Autodesk Fusion 360 part; units mm, degrees
(part 12 of 14)
  arc A3353 (43.5673, 5.334) -> (44.0627, 5.334) centre (43.815, 5.334) ccw
  line L5719 (41.91, 3.8608) -> (50.8, 3.8608)
  line L5720 (43.815, 5.08) -> (43.815, 5.588)
  line L5721 (43.561, 5.334) -> (44.069, 5.334)
  line L5722 (43.815, 5.08) -> (43.815, 5.588)
  arc A3354 (63.8873, 6.223) -> (64.3827, 6.223) centre (64.135, 6.223) ccw
  line L5723 (41.91, 6.8072) -> (41.91, 3.8608)
  line L5724 (64.389, 6.223) -> (63.881, 6.223)
  arc A3355 (64.3827, 6.223) -> (63.8873, 6.223) centre (64.135, 6.223) ccw
  arc A3356 (43.5673, 5.334) -> (44.0627, 5.334) centre (43.815, 5.334) ccw
  line L5725 (64.389, 6.223) -> (63.881, 6.223)
  arc A3357 (63.8873, 6.223) -> (64.3827, 6.223) centre (64.135, 6.223) ccw
  line L5726 (64.135, 6.477) -> (64.135, 5.969)
  line L5727 (64.135, 6.477) -> (64.135, 5.969)
  line L5728 (43.815, 5.08) -> (43.815, 5.588)
  arc A3358 (64.135, 6.477) -> (64.135, 5.969) centre (64.135, 6.223) ccw
  arc A3359 (43.5673, 5.334) -> (44.0627, 5.334) centre (43.815, 5.334) ccw
  line L5729 (43.561, 5.334) -> (44.069, 5.334)
  line L5730 (50.8, 3.8608) -> (50.8, 6.8072)
  line L5731 (43.561, 5.334) -> (44.069, 5.334)
  line L5732 (43.815, 5.08) -> (43.815, 5.588)
  arc A3360 (64.3827, 6.223) -> (63.8873, 6.223) centre (64.135, 6.223) ccw
  arc A3361 (43.5673, 5.334) -> (44.0627, 5.334) centre (43.815, 5.334) ccw
  arc A3362 (46.1073, 5.334) -> (46.6026, 5.334) centre (46.355, 5.334) ccw
  arc A3363 (46.355, 4.9403) -> (46.355, 5.7277) centre (46.355, 5.334) ccw
  arc A3364 (46.1073, 5.334) -> (46.6026, 5.334) centre (46.355, 5.334) ccw
  arc A3365 (46.6026, 5.334) -> (46.1073, 5.334) centre (46.355, 5.334) ccw
  line L5733 (46.355, 5.08) -> (46.355, 5.588)
  arc A3366 (46.355, 5.7277) -> (46.355, 4.9403) centre (46.355, 5.334) ccw
  arc A3367 (44.0627, 5.334) -> (43.5673, 5.334) centre (43.815, 5.334) ccw
  line L5734 (46.355, 5.08) -> (46.355, 5.588)
  arc A3368 (46.355, 4.9403) -> (46.355, 5.7277) centre (46.355, 5.334) ccw
  line L5735 (46.355, 5.08) -> (46.355, 5.588)
  arc A3369 (44.0627, 5.334) -> (43.5673, 5.334) centre (43.815, 5.334) ccw
  arc A3370 (46.355, 5.588) -> (46.355, 5.08) centre (46.355, 5.334) ccw
  arc A3371 (49.1427, 5.334) -> (48.6473, 5.334) centre (48.895, 5.334) ccw
  line L5736 (46.355, 5.08) -> (46.355, 5.588)
  line L5737 (43.815, 5.08) -> (43.815, 5.588)
  arc A3372 (46.1073, 5.334) -> (46.6026, 5.334) centre (46.355, 5.334) ccw
  line L5738 (46.355, 5.08) -> (46.355, 5.588)
  arc A3373 (46.1073, 5.334) -> (46.6026, 5.334) centre (46.355, 5.334) ccw
  line L5739 (43.815, 5.08) -> (43.815, 5.588)
  arc A3374 (46.6026, 5.334) -> (46.1073, 5.334) centre (46.355, 5.334) ccw
  arc A3375 (44.0627, 5.334) -> (43.5673, 5.334) centre (43.815, 5.334) ccw
  line L5740 (43.815, 5.08) -> (43.815, 5.588)
  arc A3376 (44.0627, 5.334) -> (43.5673, 5.334) centre (43.815, 5.334) ccw
  arc A3377 (48.6473, 5.334) -> (49.1427, 5.334) centre (48.895, 5.334) ccw
  arc A3378 (49.1427, 5.334) -> (48.6473, 5.334) centre (48.895, 5.334) ccw
  arc A3379 (46.6026, 5.334) -> (46.1073, 5.334) centre (46.355, 5.334) ccw
  arc A3380 (46.1073, 5.334) -> (46.6026, 5.334) centre (46.355, 5.334) ccw
  arc A3381 (46.355, 4.9403) -> (46.355, 5.7277) centre (46.355, 5.334) ccw
  arc A3382 (48.6473, 5.334) -> (49.1427, 5.334) centre (48.895, 5.334) ccw
  arc A3383 (46.1073, 5.334) -> (46.6026, 5.334) centre (46.355, 5.334) ccw
  arc A3384 (46.6026, 5.334) -> (46.1073, 5.334) centre (46.355, 5.334) ccw
  arc A3385 (46.6026, 5.334) -> (46.1073, 5.334) centre (46.355, 5.334) ccw
  arc A3386 (46.355, 5.08) -> (46.355, 5.588) centre (46.355, 5.334) ccw
  line L5741 (48.895, 5.08) -> (48.895, 5.588)
  line L5742 (46.355, 5.08) -> (46.355, 5.588)
  arc A3387 (46.6026, 5.334) -> (46.1073, 5.334) centre (46.355, 5.334) ccw
  line L5743 (46.101, 5.334) -> (46.609, 5.334)
  line L5744 (46.101, 5.334) -> (46.609, 5.334)
  line L5745 (46.101, 5.334) -> (46.609, 5.334)
  line L5746 (46.101, 5.334) -> (46.609, 5.334)
  arc A3388 (46.355, 5.7277) -> (46.355, 4.9403) centre (46.355, 5.334) ccw
  line L5747 (43.815, 5.08) -> (43.815, 5.588)
  arc A3389 (46.1073, 5.334) -> (46.6026, 5.334) centre (46.355, 5.334) ccw
  arc A3390 (46.355, 4.9403) -> (46.355, 5.7277) centre (46.355, 5.334) ccw
  arc A3391 (44.0627, 5.334) -> (43.5673, 5.334) centre (43.815, 5.334) ccw
  line L5748 (46.355, 5.08) -> (46.355, 5.588)
  arc A3392 (48.6473, 5.334) -> (49.1427, 5.334) centre (48.895, 5.334) ccw
  line L5749 (46.101, 5.334) -> (46.609, 5.334)
  line L5750 (46.101, 5.334) -> (46.609, 5.334)
  arc A3393 (46.6026, 5.334) -> (46.1073, 5.334) centre (46.355, 5.334) ccw
  arc A3394 (46.355, 5.7277) -> (46.355, 4.9403) centre (46.355, 5.334) ccw
  line L5751 (46.355, 5.08) -> (46.355, 5.588)
  arc A3395 (46.6026, 5.334) -> (46.1073, 5.334) centre (46.355, 5.334) ccw
  line L5752 (48.895, 5.08) -> (48.895, 5.588)
  arc A3396 (46.355, 4.9403) -> (46.355, 5.7277) centre (46.355, 5.334) ccw
  line L5753 (46.101, 5.334) -> (46.609, 5.334)
  line L5754 (46.101, 5.334) -> (46.609, 5.334)
  line L5755 (43.0276, 5.334) -> (44.6024, 5.334)
  arc A3397 (46.355, 5.7277) -> (46.355, 4.9403) centre (46.355, 5.334) ccw
  line L5756 (46.355, 5.08) -> (46.355, 5.588)
  arc A3398 (46.6026, 5.334) -> (46.1073, 5.334) centre (46.355, 5.334) ccw
  line L5757 (46.101, 5.334) -> (46.609, 5.334)
  line L5758 (48.641, 5.334) -> (49.149, 5.334)
  arc A3399 (46.1073, 5.334) -> (46.6026, 5.334) centre (46.355, 5.334) ccw
  arc A3400 (48.895, 4.9403) -> (48.895, 5.7277) centre (48.895, 5.334) ccw
  line L5759 (30.607, 2.667) -> (39.116, 2.667)
  arc A3401 (48.6473, 5.334) -> (49.1427, 5.334) centre (48.895, 5.334) ccw
  line L5760 (48.895, 5.08) -> (48.895, 5.588)
  line L5761 (48.895, 5.08) -> (48.895, 5.588)
  arc A3402 (46.6026, 5.334) -> (46.1073, 5.334) centre (46.355, 5.334) ccw
  arc A3403 (46.355, 5.7277) -> (46.355, 4.9403) centre (46.355, 5.334) ccw
  line L5762 (48.641, 5.334) -> (49.149, 5.334)
  arc A3404 (49.1427, 5.334) -> (48.6473, 5.334) centre (48.895, 5.334) ccw
  line L5763 (39.116, 2.667) -> (39.116, 7.747)
  arc A3405 (48.895, 5.588) -> (48.895, 5.08) centre (48.895, 5.334) ccw
  line L5764 (48.895, 5.08) -> (48.895, 5.588)
  arc A3406 (48.6473, 5.334) -> (49.1427, 5.334) centre (48.895, 5.334) ccw
  arc A3407 (49.1427, 5.334) -> (48.6473, 5.334) centre (48.895, 5.334) ccw
  arc A3408 (49.1427, 5.334) -> (48.6473, 5.334) centre (48.895, 5.334) ccw
  line L5765 (48.895, 5.08) -> (48.895, 5.588)
  arc A3409 (48.6473, 5.334) -> (49.1427, 5.334) centre (48.895, 5.334) ccw
  arc A3410 (48.895, 5.7277) -> (48.895, 4.9403) centre (48.895, 5.334) ccw
  arc A3411 (49.1427, 5.334) -> (48.6473, 5.334) centre (48.895, 5.334) ccw
  line L5766 (25.256, 2.707) -> (25.556, 3.407)
  arc A3412 (48.895, 4.9403) -> (48.895, 5.7277) centre (48.895, 5.334) ccw
  line L5767 (48.895, 5.08) -> (48.895, 5.588)
  arc A3413 (48.6473, 5.334) -> (49.1427, 5.334) centre (48.895, 5.334) ccw
  line L5768 (26.416, 6.007) -> (26.416, 8.407)
  line L5769 (26.416, 6.007) -> (26.416, 8.407)
  line L5770 (27.686, 6.007) -> (27.686, 8.407)
  arc A3414 (49.1427, 5.334) -> (48.6473, 5.334) centre (48.895, 5.334) ccw
  line L5771 (28.956, 2.007) -> (28.956, 4.407)
  line L5772 (48.641, 5.334) -> (49.149, 5.334)
  line L5773 (48.641, 5.334) -> (49.149, 5.334)
  line L5774 (48.641, 5.334) -> (49.149, 5.334)
  line L5775 (48.641, 5.334) -> (49.149, 5.334)
  arc A3415 (48.895, 5.7277) -> (48.895, 4.9403) centre (48.895, 5.334) ccw
  line L5776 (27.305, 7.747) -> (25.146, 7.747)
  arc A3416 (48.895, 4.9403) -> (48.895, 5.7277) centre (48.895, 5.334) ccw
  arc A3417 (48.895, 5.7277) -> (48.895, 4.9403) centre (48.895, 5.334) ccw
  arc A3418 (49.1427, 5.334) -> (48.6473, 5.334) centre (48.895, 5.334) ccw
  line L5777 (48.895, 5.08) -> (48.895, 5.588)
  arc A3419 (48.6473, 5.334) -> (49.1427, 5.334) centre (48.895, 5.334) ccw
  arc A3420 (48.895, 5.7277) -> (48.895, 4.9403) centre (48.895, 5.334) ccw
  arc A3421 (46.1073, 5.334) -> (46.6026, 5.334) centre (46.355, 5.334) ccw
  arc A3422 (46.1073, 5.334) -> (46.6026, 5.334) centre (46.355, 5.334) ccw
  line L5778 (48.641, 5.334) -> (49.149, 5.334)
  line L5779 (46.355, 5.08) -> (46.355, 5.588)
  line L5780 (48.895, 5.08) -> (48.895, 5.588)
  line L5781 (48.641, 5.334) -> (49.149, 5.334)
  arc A3423 (49.1427, 5.334) -> (48.6473, 5.334) centre (48.895, 5.334) ccw
  arc A3424 (48.895, 4.9403) -> (48.895, 5.7277) centre (48.895, 5.334) ccw
  arc A3425 (48.895, 4.9403) -> (48.895, 5.7277) centre (48.895, 5.334) ccw
  line L5782 (46.101, 5.334) -> (46.609, 5.334)
  line L5783 (39.116, 7.747) -> (30.607, 7.747)
  line L5784 (48.641, 5.334) -> (49.149, 5.334)
  arc A3426 (49.1427, 5.334) -> (48.6473, 5.334) centre (48.895, 5.334) ccw
  line L5785 (25.146, 7.747) -> (25.146, 2.667)
  line L5786 (25.556, 3.407) -> (25.856, 2.707)
  arc A3427 (48.895, 5.08) -> (48.895, 5.588) centre (48.895, 5.334) ccw
  line L5787 (25.146, 2.667) -> (27.305, 2.667)
  line L5788 (48.641, 5.334) -> (49.149, 5.334)
  arc A3428 (48.6473, 5.334) -> (49.1427, 5.334) centre (48.895, 5.334) ccw
  arc A3429 (48.6473, 5.334) -> (49.1427, 5.334) centre (48.895, 5.334) ccw
  arc A3430 (48.895, 5.7277) -> (48.895, 4.9403) centre (48.895, 5.334) ccw
  line L5789 (28.067, 2.667) -> (29.845, 2.667)
  line L5790 (48.895, 5.08) -> (48.895, 5.588)
  line L5791 (29.845, 7.747) -> (28.067, 7.747)
  line L5792 (36.576, 6.007) -> (36.576, 8.407)
  line L5793 (86.233, 32.893) -> (86.233, 36.703)
  line L5794 (32.766, 6.007) -> (32.766, 8.407)
  arc A3431 (85.9944, 37.338) -> (86.4716, 37.338) centre (86.233, 37.338) ccw
  line L5795 (85.344, 37.211) -> (85.852, 37.211)
  line L5796 (30.226, 2.007) -> (30.226, 4.407)
  line L5797 (34.036, 2.007) -> (34.036, 4.407)
  line L5798 (86.233, 36.703) -> (82.423, 36.703)
  line L5799 (82.804, 32.385) -> (83.312, 32.385)
  line L5800 (12.2702, 55.37) -> (18.8702, 55.37)
  line L5801 (30.226, 2.007) -> (30.226, 4.407)
  line L5802 (31.496, 2.007) -> (31.496, 4.407)
  line L5803 (30.226, 2.007) -> (30.226, 4.407)
  line L5804 (82.804, 37.211) -> (83.312, 37.211)
  line L5805 (34.036, 2.007) -> (34.036, 4.407)
  line L5806 (27.686, 6.007) -> (27.686, 8.407)
  line L5807 (35.306, 2.007) -> (35.306, 4.407)
  line L5808 (27.686, 2.007) -> (27.686, 4.407)
  line L5809 (35.306, 6.007) -> (35.306, 8.407)
  line L5810 (31.496, 6.007) -> (31.496, 8.407)
  line L5811 (35.306, 6.007) -> (35.306, 8.407)
  line L5812 (32.766, 6.007) -> (32.766, 8.407)
  line L5813 (27.686, 2.007) -> (27.686, 4.407)
  line L5814 (32.766, 2.007) -> (32.766, 4.407)
  line L5815 (34.036, 6.007) -> (34.036, 8.407)
  line L5816 (37.846, 6.007) -> (37.846, 8.407)
  line L5817 (28.956, 6.007) -> (28.956, 8.407)
  line L5818 (18.8702, 48.77) -> (12.2702, 48.77)
  line L5819 (27.686, 2.007) -> (27.686, 4.407)
  line L5820 (34.036, 6.007) -> (34.036, 8.407)
  line L5821 (82.804, 37.211) -> (83.312, 37.211)
  line L5822 (27.686, 6.007) -> (27.686, 8.407)
  line L5823 (34.036, 6.007) -> (34.036, 8.407)
  line L5824 (82.804, 32.385) -> (83.312, 32.385)
  line L5825 (84.074, 37.211) -> (84.582, 37.211)
  line L5826 (36.576, 2.007) -> (36.576, 4.407)
  line L5827 (35.306, 2.007) -> (35.306, 4.407)
  line L5828 (36.576, 6.007) -> (36.576, 8.407)
  line L5829 (28.956, 6.007) -> (28.956, 8.407)
  line L5830 (31.496, 6.007) -> (31.496, 8.407)
  line L5831 (32.766, 6.007) -> (32.766, 8.407)
  line L5832 (28.956, 2.007) -> (28.956, 4.407)
  line L5833 (36.576, 2.007) -> (36.576, 4.407)
  line L5834 (26.416, 2.007) -> (26.416, 4.407)
  line L5835 (31.496, 2.007) -> (31.496, 4.407)
  line L5836 (26.416, 2.007) -> (26.416, 4.407)
  line L5837 (30.226, 6.007) -> (30.226, 8.407)
  line L5838 (26.416, 6.007) -> (26.416, 8.407)
  line L5839 (28.956, 6.007) -> (28.956, 8.407)
  line L5840 (32.766, 2.007) -> (32.766, 4.407)
  line L5841 (30.226, 6.007) -> (30.226, 8.407)
  line L5842 (37.846, 2.007) -> (37.846, 4.407)
  line L5843 (31.496, 2.007) -> (31.496, 4.407)
  line L5844 (36.576, 2.007) -> (36.576, 4.407)
  line L5845 (34.036, 2.007) -> (34.036, 4.407)
  line L5846 (30.226, 6.007) -> (30.226, 8.407)
  line L5847 (26.416, 2.007) -> (26.416, 4.407)
  line L5848 (35.306, 2.007) -> (35.306, 4.407)
  line L5849 (36.576, 6.007) -> (36.576, 8.407)
  line L5850 (31.496, 6.007) -> (31.496, 8.407)
  line L5851 (32.766, 2.007) -> (32.766, 4.407)
  line L5852 (35.306, 6.007) -> (35.306, 8.407)
  line L5853 (85.852, 33.909) -> (85.852, 35.687)
  line L5854 (28.956, 2.007) -> (28.956, 4.407)
  line L5855 (86.106, 22.352) -> (82.296, 22.352)
  line L5856 (68.834, 38.735) -> (69.342, 38.735)
  line L5857 (82.804, 32.385) -> (83.312, 32.385)
  line L5858 (82.296, 22.352) -> (82.296, 18.542)
  line L5859 (70.104, 38.735) -> (70.612, 38.735)
  line L5860 (82.296, 18.542) -> (86.106, 18.542)
  line L5861 (18.7702, 54.27) -> (12.3702, 54.27)
  line L5862 (18.7702, 49.87) -> (12.3702, 49.87)
  arc A3432 (72.5016, 38.862) -> (72.0244, 38.862) centre (72.263, 38.862) ccw
  line L5863 (82.677, 21.336) -> (82.677, 19.558)
  line L5864 (83.185, 18.034) -> (82.677, 18.034)
  arc A3433 (86.4716, 37.338) -> (85.9944, 37.338) centre (86.233, 37.338) ccw
  line L5865 (84.074, 37.211) -> (84.582, 37.211)
  line L5866 (82.804, 35.687) -> (82.804, 33.909)
  line L5867 (72.263, 38.227) -> (68.453, 38.227)
  line L5868 (68.453, 34.417) -> (72.263, 34.417)
  line L5869 (71.374, 38.735) -> (71.882, 38.735)
  line L5870 (71.374, 33.909) -> (71.882, 33.909)
  arc A3434 (82.5346, 17.907) -> (82.0574, 17.907) centre (82.296, 17.907) ccw
  line L5871 (72.263, 34.417) -> (72.263, 38.227)
  line L5872 (82.804, 37.211) -> (83.312, 37.211)
  line L5873 (68.834, 16.764) -> (71.882, 16.764)
  line L5874 (71.882, 18.542) -> (68.834, 18.542)
  line L5875 (85.725, 18.034) -> (85.217, 18.034)
  line L5876 (71.882, 16.764) -> (71.882, 18.542)
  line L5877 (83.185, 22.86) -> (82.677, 22.86)
  line L5878 (37.846, 6.007) -> (37.846, 8.407)
  line L5879 (83.185, 18.034) -> (82.677, 18.034)
  line L5880 (68.834, 33.909) -> (69.342, 33.909)
  line L5881 (85.852, 35.687) -> (82.804, 35.687)
  line L5882 (85.344, 32.385) -> (85.852, 32.385)
  line L5883 (85.344, 32.385) -> (85.852, 32.385)
  line L5884 (82.423, 36.703) -> (82.423, 32.893)
  line L5885 (18.8702, 55.37) -> (18.8702, 48.77)
  line L5886 (84.074, 37.211) -> (84.582, 37.211)
  line L5887 (71.882, 37.211) -> (68.834, 37.211)
  line L5888 (71.374, 38.735) -> (71.882, 38.735)
  line L5889 (82.804, 33.909) -> (85.852, 33.909)
  line L5890 (70.104, 38.735) -> (70.612, 38.735)
  line L5891 (85.344, 32.385) -> (85.852, 32.385)
  line L5892 (18.7702, 54.27) -> (12.3702, 54.27)
  line L5893 (70.104, 38.735) -> (70.612, 38.735)
  line L5894 (37.846, 2.007) -> (37.846, 4.407)
  line L5895 (71.882, 35.433) -> (71.882, 37.211)
  line L5896 (68.834, 33.909) -> (69.342, 33.909)
  line L5897 (68.453, 38.227) -> (68.453, 34.417)
  line L5898 (71.374, 33.909) -> (71.882, 33.909)
  line L5899 (18.7702, 49.87) -> (12.3702, 49.87)
  arc A3435 (72.0244, 38.862) -> (72.5016, 38.862) centre (72.263, 38.862) ccw
  line L5900 (82.423, 32.893) -> (86.233, 32.893)
  line L5901 (37.846, 2.007) -> (37.846, 4.407)
  line L5902 (18.7702, 49.87) -> (12.3702, 49.87)
  line L5903 (68.834, 38.735) -> (69.342, 38.735)
  line L5904 (18.7702, 54.27) -> (12.3702, 54.27)
  line L5905 (37.846, 6.007) -> (37.846, 8.407)
  line L5906 (85.344, 37.211) -> (85.852, 37.211)
  line L5907 (68.834, 38.735) -> (69.342, 38.735)
  line L5908 (12.2702, 48.77) -> (12.2702, 55.37)
  line L5909 (85.344, 37.211) -> (85.852, 37.211)
  line L5910 (68.834, 37.211) -> (68.834, 35.433)
  line L5911 (71.374, 33.909) -> (71.882, 33.909)
  line L5912 (68.834, 33.909) -> (69.342, 33.909)
  line L5913 (71.374, 38.735) -> (71.882, 38.735)
  line L5914 (68.834, 35.433) -> (71.882, 35.433)
  line L5915 (9.652, 22.6974) -> (9.652, 24.1198)
  line L5916 (71.882, 15.24) -> (71.374, 15.24)
  line L5917 (7.659, 22.7336) -> (7.659, 24.0836)
  line L5918 (9.359, 22.7336) -> (9.359, 24.0836)
  line L5919 (69.342, 20.066) -> (68.834, 20.066)
  line L5920 (7.409, 24.1336) -> (7.409, 22.6836)
  line L5921 (85.725, 22.86) -> (85.217, 22.86)
  line L5922 (84.455, 18.034) -> (83.947, 18.034)
  line L5923 (71.882, 20.066) -> (71.374, 20.066)
  line L5924 (83.185, 22.86) -> (82.677, 22.86)
  line L5925 (7.366, 24.1198) -> (7.366, 22.6974)
  line L5926 (5.3823, 40.6654) -> (5.3823, 42.9514)
  line L5927 (85.725, 18.034) -> (85.217, 18.034)
  line L5928 (9.652, 24.1198) -> (7.366, 24.1198)
  line L5929 (3.9599, 42.9514) -> (3.9599, 40.6654)
  line L5930 (3.9599, 40.6654) -> (5.3823, 40.6654)
  line L5931 (82.677, 19.558) -> (85.725, 19.558)
  line L5932 (85.725, 18.034) -> (85.217, 18.034)
  line L5933 (5.3961, 42.9084) -> (3.9461, 42.9084)
  line L5934 (70.612, 15.24) -> (70.104, 15.24)
  line L5935 (9.652, 24.1198) -> (7.366, 24.1198)
  line L5936 (86.106, 18.542) -> (86.106, 22.352)
  line L5937 (71.882, 20.066) -> (71.374, 20.066)
  line L5938 (71.882, 15.24) -> (71.374, 15.24)
  line L5939 (7.366, 24.1198) -> (7.366, 22.6974)
  line L5940 (69.342, 20.066) -> (68.834, 20.066)
  line L5941 (71.882, 20.066) -> (71.374, 20.066)
  line L5942 (7.366, 22.6974) -> (9.652, 22.6974)
  line L5943 (9.359, 22.7336) -> (9.359, 24.0836)
  line L5944 (7.659, 22.7336) -> (7.659, 24.0836)
  line L5945 (9.609, 24.1336) -> (7.409, 24.1336)
  line L5946 (9.652, 22.6974) -> (9.652, 24.1198)
  line L5947 (7.366, 22.6974) -> (9.652, 22.6974)
  line L5948 (5.3961, 40.7084) -> (5.3961, 42.9084)
  line L5949 (85.725, 21.336) -> (82.677, 21.336)
  line L5950 (9.359, 22.7336) -> (9.359, 24.0836)
  line L5951 (3.9461, 40.7084) -> (5.3961, 40.7084)
  line L5952 (3.9461, 42.9084) -> (3.9461, 40.7084)
  line L5953 (7.659, 22.7336) -> (7.659, 24.0836)
  line L5954 (68.453, 19.558) -> (68.453, 15.748)
  line L5955 (84.455, 18.034) -> (83.947, 18.034)
  arc A3436 (68.2144, 15.113) -> (68.6916, 15.113) centre (68.453, 15.113) ccw
  line L5956 (85.725, 22.86) -> (85.217, 22.86)
  line L5957 (69.342, 15.24) -> (68.834, 15.24)
  arc A3437 (82.0574, 17.907) -> (82.5346, 17.907) centre (82.296, 17.907) ccw
  line L5958 (84.455, 18.034) -> (83.947, 18.034)
  line L5959 (69.342, 15.24) -> (68.834, 15.24)
  line L5960 (85.725, 22.86) -> (85.217, 22.86)
  line L5961 (85.725, 19.558) -> (85.725, 21.336)
  line L5962 (72.263, 15.748) -> (72.263, 19.558)
  arc A3438 (68.6916, 15.113) -> (68.2144, 15.113) centre (68.453, 15.113) ccw
  line L5963 (72.263, 19.558) -> (68.453, 19.558)
  line L5964 (68.453, 15.748) -> (72.263, 15.748)
  line L5965 (83.185, 22.86) -> (82.677, 22.86)
  line L5966 (83.185, 18.034) -> (82.677, 18.034)
  line L5967 (7.409, 22.6836) -> (9.609, 22.6836)
  line L5968 (71.882, 15.24) -> (71.374, 15.24)
  line L5969 (68.834, 18.542) -> (68.834, 16.764)
  line L5970 (9.609, 22.6836) -> (9.609, 24.1336)
  line L5971 (5.3823, 42.9514) -> (3.9599, 42.9514)
  line L5972 (70.612, 15.24) -> (70.104, 15.24)
  line L5973 (70.612, 15.24) -> (70.104, 15.24)
  line L5974 (69.342, 20.066) -> (68.834, 20.066)
  line L5975 (69.342, 15.24) -> (68.834, 15.24)
  arc A3439 (93.345, 58.039) -> (93.345, 58.801) centre (93.345, 58.42) ccw
  arc A3440 (93.0973, 58.42) -> (93.5927, 58.42) centre (93.345, 58.42) ccw
  arc A3441 (93.345, 58.801) -> (93.345, 58.039) centre (93.345, 58.42) ccw
  arc A3442 (93.345, 58.801) -> (93.345, 58.039) centre (93.345, 58.42) ccw
  arc A3443 (74.4157, 6.858) -> (73.9203, 6.858) centre (74.168, 6.858) ccw
  line L5976 (23.218, 39.551) -> (16.818, 39.551)
  arc A3444 (93.5927, 58.42) -> (93.0973, 58.42) centre (93.345, 58.42) ccw
  line L5977 (93.091, 58.42) -> (93.599, 58.42)
  line L5978 (93.091, 58.42) -> (93.599, 58.42)
  line L5979 (93.345, 58.166) -> (93.345, 58.674)
  line L5980 (16.718, 45.051) -> (23.318, 45.051)
  arc A3445 (74.168, 7.493) -> (74.168, 6.223) centre (74.168, 6.858) ccw
  line L5981 (93.345, 58.166) -> (93.345, 58.674)
  arc A3446 (74.4157, 6.858) -> (73.9203, 6.858) centre (74.168, 6.858) ccw
  arc A3447 (93.345, 59.055) -> (93.345, 57.785) centre (93.345, 58.42) ccw
  line L5982 (93.091, 58.42) -> (93.599, 58.42)
  arc A3448 (94.615, 58.42) -> (92.075, 58.42) centre (93.345, 58.42) ccw
  arc A3449 (93.0973, 58.42) -> (93.5927, 58.42) centre (93.345, 58.42) ccw
  line L5983 (93.345, 58.166) -> (93.345, 58.674)
  arc A3450 (94.5919, 58.42) -> (92.0981, 58.42) centre (93.345, 58.42) ccw
  line L5984 (93.345, 58.166) -> (93.345, 58.674)
  line L5985 (3.9599, 42.9514) -> (3.9599, 40.6654)
  line L5986 (5.3461, 40.9584) -> (3.9961, 40.9584)
  line L5987 (93.091, 58.42) -> (93.599, 58.42)
  line L5988 (93.091, 58.42) -> (93.599, 58.42)
  line L5989 (93.345, 58.166) -> (93.345, 58.674)
  arc A3451 (93.5927, 58.42) -> (93.0973, 58.42) centre (93.345, 58.42) ccw
  arc A3452 (72.9211, 6.858) -> (75.4149, 6.858) centre (74.168, 6.858) ccw
  arc A3453 (93.5927, 58.42) -> (93.0973, 58.42) centre (93.345, 58.42) ccw
  line L5990 (5.3461, 42.6584) -> (3.9961, 42.6584)
  line L5991 (5.3461, 40.9584) -> (3.9961, 40.9584)
  line L5992 (23.218, 39.551) -> (16.818, 39.551)
  line L5993 (23.218, 39.551) -> (16.818, 39.551)
  arc A3454 (93.0973, 58.42) -> (93.5927, 58.42) centre (93.345, 58.42) ccw
  arc A3455 (93.0973, 58.42) -> (93.5927, 58.42) centre (93.345, 58.42) ccw
  arc A3456 (92.0981, 58.42) -> (94.5919, 58.42) centre (93.345, 58.42) ccw
  line L5994 (74.168, 7.112) -> (74.168, 6.604)
  line L5995 (5.3461, 40.9584) -> (3.9961, 40.9584)
  arc A3457 (92.075, 58.42) -> (94.615, 58.42) centre (93.345, 58.42) ccw
  arc A3458 (93.5927, 58.42) -> (93.0973, 58.42) centre (93.345, 58.42) ccw
  line L5996 (23.218, 43.951) -> (16.818, 43.951)
  arc A3459 (93.0973, 58.42) -> (93.5927, 58.42) centre (93.345, 58.42) ccw
  line L5997 (93.345, 58.166) -> (93.345, 58.674)
  line L5998 (5.3823, 42.9514) -> (3.9599, 42.9514)
  line L5999 (5.3823, 40.6654) -> (5.3823, 42.9514)
  line L6000 (5.3461, 42.6584) -> (3.9961, 42.6584)
  line L6001 (5.3461, 42.6584) -> (3.9961, 42.6584)
  line L6002 (23.218, 43.951) -> (16.818, 43.951)
  line L6003 (23.218, 43.951) -> (16.818, 43.951)
  line L6004 (74.422, 6.858) -> (73.914, 6.858)
  line L6005 (16.718, 38.451) -> (16.718, 45.051)
  line L6006 (23.318, 38.451) -> (16.718, 38.451)
  line L6007 (3.9599, 40.6654) -> (5.3823, 40.6654)
  line L6008 (93.091, 58.42) -> (93.599, 58.42)
  line L6009 (93.091, 58.42) -> (93.599, 58.42)
  arc A3460 (93.345, 58.039) -> (93.345, 58.801) centre (93.345, 58.42) ccw
  line L6010 (93.345, 58.166) -> (93.345, 58.674)
  arc A3461 (93.345, 57.785) -> (93.345, 59.055) centre (93.345, 58.42) ccw
  line L6011 (23.318, 45.051) -> (23.318, 38.451)
  line L6012 (74.422, 6.858) -> (73.914, 6.858)
  arc A3462 (93.0973, 58.42) -> (93.5927, 58.42) centre (93.345, 58.42) ccw
  line L6013 (93.345, 58.166) -> (93.345, 58.674)
  arc A3463 (74.168, 6.223) -> (74.168, 7.493) centre (74.168, 6.858) ccw
  arc A3464 (93.5927, 58.42) -> (93.0973, 58.42) centre (93.345, 58.42) ccw
  arc A3465 (74.168, 7.239) -> (74.168, 6.477) centre (74.168, 6.858) ccw
  line L6014 (74.168, 7.112) -> (74.168, 6.604)
  arc A3466 (74.168, 6.477) -> (74.168, 7.239) centre (74.168, 6.858) ccw
  arc A3467 (74.4157, 6.858) -> (73.9203, 6.858) centre (74.168, 6.858) ccw
  arc A3468 (73.9203, 6.858) -> (74.4157, 6.858) centre (74.168, 6.858) ccw
  arc A3469 (74.168, 6.477) -> (74.168, 7.239) centre (74.168, 6.858) ccw
  arc A3470 (75.4149, 6.858) -> (72.9211, 6.858) centre (74.168, 6.858) ccw
  line L6015 (93.345, 58.166) -> (93.345, 58.674)
  arc A3471 (92.4623, 3.175) -> (92.9577, 3.175) centre (92.71, 3.175) ccw
  line L6016 (74.422, 6.858) -> (73.914, 6.858)
  line L6017 (74.422, 6.858) -> (73.914, 6.858)
  arc A3472 (92.71, 3.81) -> (92.71, 2.54) centre (92.71, 3.175) ccw
  line L6018 (74.168, 7.112) -> (74.168, 6.604)
  arc A3473 (74.168, 7.239) -> (74.168, 6.477) centre (74.168, 6.858) ccw
  arc A3474 (92.71, 2.54) -> (92.71, 3.81) centre (92.71, 3.175) ccw
  arc A3475 (73.9203, 6.858) -> (74.4157, 6.858) centre (74.168, 6.858) ccw
  arc A3476 (93.0973, 58.42) -> (93.5927, 58.42) centre (93.345, 58.42) ccw
  arc A3477 (93.345, 58.801) -> (93.345, 58.039) centre (93.345, 58.42) ccw
  line L6019 (74.422, 6.858) -> (73.914, 6.858)
  line L6020 (92.71, 2.921) -> (92.71, 3.429)
  line L6021 (74.422, 6.858) -> (73.914, 6.858)
  arc A3478 (93.345, 58.801) -> (93.345, 58.039) centre (93.345, 58.42) ccw
  arc A3479 (93.345, 58.039) -> (93.345, 58.801) centre (93.345, 58.42) ccw
  arc A3480 (74.168, 7.239) -> (74.168, 6.477) centre (74.168, 6.858) ccw
  arc A3481 (74.168, 6.477) -> (74.168, 7.239) centre (74.168, 6.858) ccw
  line L6022 (74.168, 7.112) -> (74.168, 6.604)
  arc A3482 (92.9577, 3.175) -> (92.4623, 3.175) centre (92.71, 3.175) ccw
  line L6023 (92.456, 3.175) -> (92.964, 3.175)
  arc A3483 (93.5927, 58.42) -> (93.0973, 58.42) centre (93.345, 58.42) ccw
  arc A3484 (73.9203, 6.858) -> (74.4157, 6.858) centre (74.168, 6.858) ccw
  line L6024 (74.422, 6.858) -> (73.914, 6.858)
  arc A3485 (93.5927, 58.42) -> (93.0973, 58.42) centre (93.345, 58.42) ccw
  line L6025 (74.168, 7.112) -> (74.168, 6.604)
  arc A3486 (74.168, 7.239) -> (74.168, 6.477) centre (74.168, 6.858) ccw
  arc A3487 (74.4157, 6.858) -> (73.9203, 6.858) centre (74.168, 6.858) ccw
  line L6026 (93.091, 58.42) -> (93.599, 58.42)
  arc A3488 (73.9203, 6.858) -> (74.4157, 6.858) centre (74.168, 6.858) ccw
  arc A3489 (92.4623, 3.175) -> (92.9577, 3.175) centre (92.71, 3.175) ccw
  arc A3490 (74.4157, 6.858) -> (73.9203, 6.858) centre (74.168, 6.858) ccw
  arc A3491 (93.345, 58.039) -> (93.345, 58.801) centre (93.345, 58.42) ccw
  arc A3492 (93.0973, 58.42) -> (93.5927, 58.42) centre (93.345, 58.42) ccw
  line L6027 (93.091, 58.42) -> (93.599, 58.42)
  arc A3493 (73.9203, 6.858) -> (74.4157, 6.858) centre (74.168, 6.858) ccw
  arc A3494 (93.0973, 58.42) -> (93.5927, 58.42) centre (93.345, 58.42) ccw
  arc A3495 (93.5927, 58.42) -> (93.0973, 58.42) centre (93.345, 58.42) ccw
  arc A3496 (93.0973, 58.42) -> (93.5927, 58.42) centre (93.345, 58.42) ccw
  arc A3497 (93.345, 58.039) -> (93.345, 58.801) centre (93.345, 58.42) ccw
  line L6028 (74.422, 6.858) -> (73.914, 6.858)
  arc A3498 (93.5927, 58.42) -> (93.0973, 58.42) centre (93.345, 58.42) ccw
  arc A3499 (74.4157, 6.858) -> (73.9203, 6.858) centre (74.168, 6.858) ccw
  line L6029 (74.168, 7.112) -> (74.168, 6.604)
  line L6030 (93.345, 58.166) -> (93.345, 58.674)
  arc A3500 (73.9203, 6.858) -> (74.4157, 6.858) centre (74.168, 6.858) ccw
  arc A3501 (73.9203, 6.858) -> (74.4157, 6.858) centre (74.168, 6.858) ccw
  arc A3502 (74.4157, 6.858) -> (73.9203, 6.858) centre (74.168, 6.858) ccw
  arc A3503 (75.438, 6.858) -> (72.898, 6.858) centre (74.168, 6.858) ccw
  arc A3504 (72.898, 6.858) -> (75.438, 6.858) centre (74.168, 6.858) ccw
  arc A3505 (93.5927, 58.42) -> (93.0973, 58.42) centre (93.345, 58.42) ccw
  arc A3506 (92.4623, 3.175) -> (92.9577, 3.175) centre (92.71, 3.175) ccw
  line L6031 (93.091, 58.42) -> (93.599, 58.42)
  line L6032 (74.422, 6.858) -> (73.914, 6.858)
  arc A3507 (93.345, 58.801) -> (93.345, 58.039) centre (93.345, 58.42) ccw
  arc A3508 (92.9577, 3.175) -> (92.4623, 3.175) centre (92.71, 3.175) ccw
  line L6033 (74.168, 7.112) -> (74.168, 6.604)
  arc A3509 (92.9577, 3.175) -> (92.4623, 3.175) centre (92.71, 3.175) ccw
  arc A3510 (80.2703, 5.715) -> (80.7657, 5.715) centre (80.518, 5.715) ccw
  arc A3511 (73.9203, 6.858) -> (74.4157, 6.858) centre (74.168, 6.858) ccw
  line L6034 (80.772, 5.715) -> (80.264, 5.715)
  line L6035 (80.518, 5.969) -> (80.518, 5.461)
  arc A3512 (74.4157, 6.858) -> (73.9203, 6.858) centre (74.168, 6.858) ccw
  arc A3513 (74.4157, 6.858) -> (73.9203, 6.858) centre (74.168, 6.858) ccw
  line L6036 (74.168, 7.112) -> (74.168, 6.604)
  line L6037 (92.71, 2.921) -> (92.71, 3.429)
  line L6038 (92.456, 3.175) -> (92.964, 3.175)
  arc A3514 (92.71, 2.794) -> (92.71, 3.556) centre (92.71, 3.175) ccw
  arc A3515 (81.788, 5.715) -> (79.248, 5.715) centre (80.518, 5.715) ccw
  line L6039 (80.518, 5.969) -> (80.518, 5.461)
  arc A3516 (92.71, 3.556) -> (92.71, 2.794) centre (92.71, 3.175) ccw
  arc A3517 (73.9203, 6.858) -> (74.4157, 6.858) centre (74.168, 6.858) ccw
  line L6040 (74.168, 7.112) -> (74.168, 6.604)
  line L6041 (80.772, 5.715) -> (80.264, 5.715)
  arc A3518 (80.518, 5.08) -> (80.518, 6.35) centre (80.518, 5.715) ccw
  line L6042 (92.71, 2.921) -> (92.71, 3.429)
  line L6043 (92.456, 3.175) -> (92.964, 3.175)
  arc A3519 (92.4623, 3.175) -> (92.9577, 3.175) centre (92.71, 3.175) ccw
  arc A3520 (91.44, 3.175) -> (93.98, 3.175) centre (92.71, 3.175) ccw
  arc A3521 (92.4623, 3.175) -> (92.9577, 3.175) centre (92.71, 3.175) ccw
  line L6044 (92.456, 3.175) -> (92.964, 3.175)
  arc A3522 (92.9577, 3.175) -> (92.4623, 3.175) centre (92.71, 3.175) ccw
  line L6045 (92.456, 3.175) -> (92.964, 3.175)
  arc A3523 (80.7657, 5.715) -> (80.2703, 5.715) centre (80.518, 5.715) ccw
  arc A3524 (92.71, 3.556) -> (92.71, 2.794) centre (92.71, 3.175) ccw
  arc A3525 (92.9577, 3.175) -> (92.4623, 3.175) centre (92.71, 3.175) ccw
  arc A3526 (92.71, 3.556) -> (92.71, 2.794) centre (92.71, 3.175) ccw
  arc A3527 (92.4623, 3.175) -> (92.9577, 3.175) centre (92.71, 3.175) ccw
  line L6046 (80.518, 5.969) -> (80.518, 5.461)
  arc A3528 (80.7657, 5.715) -> (80.2703, 5.715) centre (80.518, 5.715) ccw
  line L6047 (92.71, 2.921) -> (92.71, 3.429)
  line L6048 (92.71, 2.921) -> (92.71, 3.429)
  arc A3529 (92.9577, 3.175) -> (92.4623, 3.175) centre (92.71, 3.175) ccw
  arc A3530 (73.9203, 6.858) -> (74.4157, 6.858) centre (74.168, 6.858) ccw
  line L6049 (74.422, 6.858) -> (73.914, 6.858)
  line L6050 (74.168, 7.112) -> (74.168, 6.604)
  arc A3531 (91.4631, 3.175) -> (93.9569, 3.175) centre (92.71, 3.175) ccw
  line L6051 (92.71, 2.921) -> (92.71, 3.429)
  line L6052 (92.456, 3.175) -> (92.964, 3.175)
  line L6053 (92.456, 3.175) -> (92.964, 3.175)
  arc A3532 (74.168, 7.239) -> (74.168, 6.477) centre (74.168, 6.858) ccw
  arc A3533 (93.9569, 3.175) -> (91.4631, 3.175) centre (92.71, 3.175) ccw
  arc A3534 (74.4157, 6.858) -> (73.9203, 6.858) centre (74.168, 6.858) ccw
  arc A3535 (92.4623, 3.175) -> (92.9577, 3.175) centre (92.71, 3.175) ccw
  arc A3536 (74.168, 6.477) -> (74.168, 7.239) centre (74.168, 6.858) ccw
  arc A3537 (74.168, 6.477) -> (74.168, 7.239) centre (74.168, 6.858) ccw
  line L6054 (92.71, 2.921) -> (92.71, 3.429)
  arc A3538 (93.98, 3.175) -> (91.44, 3.175) centre (92.71, 3.175) ccw
  line L6055 (80.772, 5.715) -> (80.264, 5.715)
  line L6056 (92.456, 3.175) -> (92.964, 3.175)
  arc A3539 (92.9577, 3.175) -> (92.4623, 3.175) centre (92.71, 3.175) ccw
  arc A3540 (92.71, 2.794) -> (92.71, 3.556) centre (92.71, 3.175) ccw
  arc A3541 (81.7649, 5.715) -> (79.2711, 5.715) centre (80.518, 5.715) ccw
  arc A3542 (80.518, 6.35) -> (80.518, 5.08) centre (80.518, 5.715) ccw
  arc A3543 (92.9577, 3.175) -> (92.4623, 3.175) centre (92.71, 3.175) ccw
  arc A3544 (92.71, 2.794) -> (92.71, 3.556) centre (92.71, 3.175) ccw
  arc A3545 (80.7657, 5.715) -> (80.2703, 5.715) centre (80.518, 5.715) ccw
  line L6057 (92.456, 3.175) -> (92.964, 3.175)
  arc A3546 (80.7657, 5.715) -> (80.2703, 5.715) centre (80.518, 5.715) ccw
  arc A3547 (79.2711, 5.715) -> (81.7649, 5.715) centre (80.518, 5.715) ccw
  line L6058 (80.772, 5.715) -> (80.264, 5.715)
  line L6059 (80.518, 5.969) -> (80.518, 5.461)
  line L6060 (80.772, 5.715) -> (80.264, 5.715)
  arc A3548 (80.2703, 5.715) -> (80.7657, 5.715) centre (80.518, 5.715) ccw
  arc A3549 (80.2703, 5.715) -> (80.7657, 5.715) centre (80.518, 5.715) ccw
  arc A3550 (84.0677, 5.588) -> (83.5724, 5.588) centre (83.82, 5.588) ccw
  line L6061 (84.074, 5.588) -> (83.566, 5.588)
  arc A3551 (80.2703, 5.715) -> (80.7657, 5.715) centre (80.518, 5.715) ccw
  line L6062 (80.518, 5.969) -> (80.518, 5.461)
  arc A3552 (80.518, 6.096) -> (80.518, 5.334) centre (80.518, 5.715) ccw
  line L6063 (80.772, 5.715) -> (80.264, 5.715)
  line L6064 (92.71, 2.921) -> (92.71, 3.429)
  arc A3553 (92.9577, 3.175) -> (92.4623, 3.175) centre (92.71, 3.175) ccw
  arc A3554 (80.518, 6.096) -> (80.518, 5.334) centre (80.518, 5.715) ccw
  arc A3555 (80.7657, 5.715) -> (80.2703, 5.715) centre (80.518, 5.715) ccw
  arc A3556 (80.7657, 5.715) -> (80.2703, 5.715) centre (80.518, 5.715) ccw
  line L6065 (92.71, 2.921) -> (92.71, 3.429)
  arc A3557 (92.4623, 3.175) -> (92.9577, 3.175) centre (92.71, 3.175) ccw
  line L6066 (80.518, 5.969) -> (80.518, 5.461)
  arc A3558 (80.2703, 5.715) -> (80.7657, 5.715) centre (80.518, 5.715) ccw
  arc A3559 (80.518, 6.096) -> (80.518, 5.334) centre (80.518, 5.715) ccw
  line L6067 (83.82, 5.842) -> (83.82, 5.334)
  arc A3560 (83.82, 4.953) -> (83.82, 6.223) centre (83.82, 5.588) ccw
  arc A3561 (80.2703, 5.715) -> (80.7657, 5.715) centre (80.518, 5.715) ccw
  arc A3562 (80.7657, 5.715) -> (80.2703, 5.715) centre (80.518, 5.715) ccw
  arc A3563 (84.0677, 5.588) -> (83.5724, 5.588) centre (83.82, 5.588) ccw
  arc A3564 (82.55, 5.588) -> (85.09, 5.588) centre (83.82, 5.588) ccw
  arc A3565 (80.7657, 5.715) -> (80.2703, 5.715) centre (80.518, 5.715) ccw
  arc A3566 (82.5731, 5.588) -> (85.0669, 5.588) centre (83.82, 5.588) ccw
  arc A3567 (83.5724, 5.588) -> (84.0677, 5.588) centre (83.82, 5.588) ccw
  arc A3568 (83.5724, 5.588) -> (84.0677, 5.588) centre (83.82, 5.588) ccw
  line L6068 (83.82, 5.842) -> (83.82, 5.334)
  arc A3569 (79.248, 5.715) -> (81.788, 5.715) centre (80.518, 5.715) ccw
  arc A3570 (83.5724, 5.588) -> (84.0677, 5.588) centre (83.82, 5.588) ccw
  arc A3571 (84.0677, 5.588) -> (83.5724, 5.588) centre (83.82, 5.588) ccw
  arc A3572 (80.518, 5.334) -> (80.518, 6.096) centre (80.518, 5.715) ccw
  arc A3573 (92.4623, 3.175) -> (92.9577, 3.175) centre (92.71, 3.175) ccw
  line L6069 (84.074, 5.588) -> (83.566, 5.588)
  line L6070 (84.074, 5.588) -> (83.566, 5.588)
  line L6071 (92.71, 2.921) -> (92.71, 3.429)
  arc A3574 (84.0677, 5.588) -> (83.5724, 5.588) centre (83.82, 5.588) ccw
  line L6072 (80.518, 5.969) -> (80.518, 5.461)
  line L6073 (80.772, 5.715) -> (80.264, 5.715)
  arc A3575 (80.518, 5.334) -> (80.518, 6.096) centre (80.518, 5.715) ccw
  arc A3576 (92.9577, 3.175) -> (92.4623, 3.175) centre (92.71, 3.175) ccw
  arc A3577 (92.71, 2.794) -> (92.71, 3.556) centre (92.71, 3.175) ccw
  arc A3578 (92.4623, 3.175) -> (92.9577, 3.175) centre (92.71, 3.175) ccw
  arc A3579 (80.2703, 5.715) -> (80.7657, 5.715) centre (80.518, 5.715) ccw
  line L6074 (84.074, 5.588) -> (83.566, 5.588)
  line L6075 (80.772, 5.715) -> (80.264, 5.715)
  arc A3580 (80.518, 6.096) -> (80.518, 5.334) centre (80.518, 5.715) ccw
  arc A3581 (85.0669, 5.588) -> (82.5731, 5.588) centre (83.82, 5.588) ccw
  arc A3582 (80.518, 6.096) -> (80.518, 5.334) centre (80.518, 5.715) ccw
  arc A3583 (92.71, 3.556) -> (92.71, 2.794) centre (92.71, 3.175) ccw
  arc A3584 (85.09, 5.588) -> (82.55, 5.588) centre (83.82, 5.588) ccw
  arc A3585 (92.71, 3.556) -> (92.71, 2.794) centre (92.71, 3.175) ccw
  arc A3586 (92.71, 2.794) -> (92.71, 3.556) centre (92.71, 3.175) ccw
  arc A3587 (83.82, 6.223) -> (83.82, 4.953) centre (83.82, 5.588) ccw
  line L6076 (83.82, 5.842) -> (83.82, 5.334)
  line L6077 (80.518, 5.969) -> (80.518, 5.461)
  line L6078 (92.456, 3.175) -> (92.964, 3.175)
  line L6079 (80.772, 5.715) -> (80.264, 5.715)
  arc A3588 (80.2703, 5.715) -> (80.7657, 5.715) centre (80.518, 5.715) ccw
  line L6080 (80.772, 5.715) -> (80.264, 5.715)
  arc A3589 (84.0677, 5.588) -> (83.5724, 5.588) centre (83.82, 5.588) ccw
  line L6081 (83.82, 5.842) -> (83.82, 5.334)
  line L6082 (80.518, 5.969) -> (80.518, 5.461)
  arc A3590 (77.216, 5.08) -> (77.216, 6.35) centre (77.216, 5.715) ccw
  arc A3591 (83.5724, 5.588) -> (84.0677, 5.588) centre (83.82, 5.588) ccw
  arc A3592 (77.216, 6.35) -> (77.216, 5.08) centre (77.216, 5.715) ccw
  arc A3593 (78.486, 5.715) -> (75.946, 5.715) centre (77.216, 5.715) ccw
  arc A3594 (84.0677, 5.588) -> (83.5724, 5.588) centre (83.82, 5.588) ccw
  arc A3595 (83.5724, 5.588) -> (84.0677, 5.588) centre (83.82, 5.588) ccw
  arc A3596 (77.4637, 5.715) -> (76.9684, 5.715) centre (77.216, 5.715) ccw
  arc A3597 (84.0677, 5.588) -> (83.5724, 5.588) centre (83.82, 5.588) ccw
  line L6083 (77.47, 5.715) -> (76.962, 5.715)
  line L6084 (77.47, 5.715) -> (76.962, 5.715)
  line L6085 (83.82, 5.842) -> (83.82, 5.334)
  line L6086 (83.82, 5.842) -> (83.82, 5.334)
  arc A3598 (83.82, 5.207) -> (83.82, 5.969) centre (83.82, 5.588) ccw
  line L6087 (77.47, 5.715) -> (76.962, 5.715)
  arc A3599 (80.518, 5.334) -> (80.518, 6.096) centre (80.518, 5.715) ccw
  arc A3600 (83.82, 5.207) -> (83.82, 5.969) centre (83.82, 5.588) ccw
  arc A3601 (83.82, 5.969) -> (83.82, 5.207) centre (83.82, 5.588) ccw
  arc A3602 (76.9684, 5.715) -> (77.4637, 5.715) centre (77.216, 5.715) ccw
  arc A3603 (80.2703, 5.715) -> (80.7657, 5.715) centre (80.518, 5.715) ccw
  arc A3604 (83.82, 5.969) -> (83.82, 5.207) centre (83.82, 5.588) ccw
  arc A3605 (76.9684, 5.715) -> (77.4637, 5.715) centre (77.216, 5.715) ccw
  line L6088 (77.216, 5.969) -> (77.216, 5.461)
  line L6089 (84.074, 5.588) -> (83.566, 5.588)
  arc A3606 (84.0677, 5.588) -> (83.5724, 5.588) centre (83.82, 5.588) ccw
  arc A3607 (84.0677, 5.588) -> (83.5724, 5.588) centre (83.82, 5.588) ccw
  arc A3608 (83.5724, 5.588) -> (84.0677, 5.588) centre (83.82, 5.588) ccw
  arc A3609 (83.5724, 5.588) -> (84.0677, 5.588) centre (83.82, 5.588) ccw
  arc A3610 (75.946, 5.715) -> (78.486, 5.715) centre (77.216, 5.715) ccw
  arc A3611 (80.2703, 5.715) -> (80.7657, 5.715) centre (80.518, 5.715) ccw
  arc A3612 (80.7657, 5.715) -> (80.2703, 5.715) centre (80.518, 5.715) ccw
  arc A3613 (83.82, 5.207) -> (83.82, 5.969) centre (83.82, 5.588) ccw
  arc A3614 (83.82, 5.207) -> (83.82, 5.969) centre (83.82, 5.588) ccw
  line L6090 (84.074, 5.588) -> (83.566, 5.588)
  arc A3615 (84.0677, 5.588) -> (83.5724, 5.588) centre (83.82, 5.588) ccw
  arc A3616 (76.9684, 5.715) -> (77.4637, 5.715) centre (77.216, 5.715) ccw
  line L6091 (77.47, 5.715) -> (76.962, 5.715)
  line L6092 (77.216, 5.969) -> (77.216, 5.461)
  arc A3617 (77.4637, 5.715) -> (76.9684, 5.715) centre (77.216, 5.715) ccw
  arc A3618 (80.518, 5.334) -> (80.518, 6.096) centre (80.518, 5.715) ccw
  arc A3619 (83.82, 5.207) -> (83.82, 5.969) centre (83.82, 5.588) ccw
  arc A3620 (83.82, 5.969) -> (83.82, 5.207) centre (83.82, 5.588) ccw
  arc A3621 (80.7657, 5.715) -> (80.2703, 5.715) centre (80.518, 5.715) ccw
  line L6093 (80.518, 5.969) -> (80.518, 5.461)
  arc A3622 (75.9691, 5.715) -> (78.4629, 5.715) centre (77.216, 5.715) ccw
  arc A3623 (77.4637, 5.715) -> (76.9684, 5.715) centre (77.216, 5.715) ccw
  arc A3624 (80.518, 5.334) -> (80.518, 6.096) centre (80.518, 5.715) ccw
  arc A3625 (77.4637, 5.715) -> (76.9684, 5.715) centre (77.216, 5.715) ccw
  line L6094 (83.82, 5.842) -> (83.82, 5.334)
  arc A3626 (83.82, 5.969) -> (83.82, 5.207) centre (83.82, 5.588) ccw
  line L6095 (77.216, 5.969) -> (77.216, 5.461)
  line L6096 (83.82, 5.842) -> (83.82, 5.334)
  line L6097 (84.074, 5.588) -> (83.566, 5.588)
  arc A3627 (83.5724, 5.588) -> (84.0677, 5.588) centre (83.82, 5.588) ccw
  arc A3628 (83.5724, 5.588) -> (84.0677, 5.588) centre (83.82, 5.588) ccw
  line L6098 (84.074, 5.588) -> (83.566, 5.588)
  arc A3629 (83.5724, 5.588) -> (84.0677, 5.588) centre (83.82, 5.588) ccw
  line L6099 (83.82, 5.842) -> (83.82, 5.334)
  arc A3630 (78.4629, 5.715) -> (75.9691, 5.715) centre (77.216, 5.715) ccw
  line L6100 (77.216, 5.969) -> (77.216, 5.461)
  line L6101 (84.074, 5.588) -> (83.566, 5.588)
  line L6102 (83.82, 5.842) -> (83.82, 5.334)
  arc A3631 (76.9684, 5.715) -> (77.4637, 5.715) centre (77.216, 5.715) ccw
  arc A3632 (85.852, 29.718) -> (85.852, 30.226) centre (85.852, 29.972) ccw
  line L6103 (94.2086, 32.9184) -> (94.2086, 34.8996)
  line L6104 (94.2086, 34.8996) -> (92.2274, 34.8996)
  arc A3633 (76.9684, 5.715) -> (77.4637, 5.715) centre (77.216, 5.715) ccw
  arc A3634 (78.873, 22.6129) -> (78.873, 22.4351) centre (78.873, 22.524) ccw
  arc A3635 (77.216, 5.334) -> (77.216, 6.096) centre (77.216, 5.715) ccw
  line L6105 (91.948, 33.274) -> (92.583, 32.639)
  line L6106 (92.71, 35.4076) -> (93.726, 35.4076)
  line L6107 (94.7166, 32.8041) -> (94.7166, 35.0139)
  arc A3636 (80.473, 22.6129) -> (80.473, 22.4351) centre (80.473, 22.524) ccw
  arc A3637 (77.4637, 5.715) -> (76.9684, 5.715) centre (77.216, 5.715) ccw
  line L6108 (77.216, 5.969) -> (77.216, 5.461)
  arc A3638 (76.9684, 5.715) -> (77.4637, 5.715) centre (77.216, 5.715) ccw
  line L6109 (91.7194, 32.8041) -> (91.7194, 35.0139)
  line L6110 (70.673, 21.524) -> (70.673, 32.324)
  arc A3639 (77.216, 5.334) -> (77.216, 6.096) centre (77.216, 5.715) ccw
  arc A3640 (85.852, 30.226) -> (85.852, 29.718) centre (85.852, 29.972) ccw
  arc A3641 (85.344, 29.972) -> (86.36, 29.972) centre (85.852, 29.972) ccw
  arc A3642 (77.216, 6.096) -> (77.216, 5.334) centre (77.216, 5.715) ccw
  line L6111 (94.488, 32.639) -> (94.488, 35.179)
  arc A3643 (77.4637, 5.715) -> (76.9684, 5.715) centre (77.216, 5.715) ccw
  line L6112 (77.216, 5.969) -> (77.216, 5.461)
  arc A3644 (76.9684, 5.715) -> (77.4637, 5.715) centre (77.216, 5.715) ccw
  line L6113 (77.47, 5.715) -> (76.962, 5.715)
  arc A3645 (85.852, 29.718) -> (85.852, 30.226) centre (85.852, 29.972) ccw
  arc A3646 (77.216, 6.096) -> (77.216, 5.334) centre (77.216, 5.715) ccw
  arc A3647 (86.36, 29.972) -> (85.344, 29.972) centre (85.852, 29.972) ccw
  arc A3648 (78.873, 22.4351) -> (78.873, 22.6129) centre (78.873, 22.524) ccw
  arc A3649 (77.4637, 5.715) -> (76.9684, 5.715) centre (77.216, 5.715) ccw
  arc A3650 (79.673, 22.6129) -> (79.673, 22.4351) centre (79.673, 22.524) ccw
  line L6114 (92.71, 32.4104) -> (93.726, 32.4104)
  line L6115 (77.47, 5.715) -> (76.962, 5.715)
  arc A3651 (77.4637, 5.715) -> (76.9684, 5.715) centre (77.216, 5.715) ccw
  line L6116 (77.216, 5.969) -> (77.216, 5.461)
  line L6117 (91.7194, 32.8041) -> (91.7194, 35.0139)
  line L6118 (77.216, 5.969) -> (77.216, 5.461)
  line L6119 (92.2274, 34.8996) -> (92.2274, 32.9184)
  arc A3652 (80.473, 22.4351) -> (80.473, 22.6129) centre (80.473, 22.524) ccw
  arc A3653 (85.344, 29.972) -> (86.36, 29.972) centre (85.852, 29.972) ccw
  line L6120 (77.47, 5.715) -> (76.962, 5.715)
  arc A3654 (77.216, 5.334) -> (77.216, 6.096) centre (77.216, 5.715) ccw
  arc A3655 (77.216, 6.096) -> (77.216, 5.334) centre (77.216, 5.715) ccw
  line L6121 (91.948, 35.179) -> (91.948, 33.274)
  arc A3656 (77.216, 6.096) -> (77.216, 5.334) centre (77.216, 5.715) ccw
  arc A3657 (83.82, 5.969) -> (83.82, 5.207) centre (83.82, 5.588) ccw
  line L6122 (84.074, 5.588) -> (83.566, 5.588)
  arc A3658 (77.4637, 5.715) -> (76.9684, 5.715) centre (77.216, 5.715) ccw
  line L6123 (77.47, 5.715) -> (76.962, 5.715)
  arc A3659 (77.4637, 5.715) -> (76.9684, 5.715) centre (77.216, 5.715) ccw
  arc A3660 (76.9684, 5.715) -> (77.4637, 5.715) centre (77.216, 5.715) ccw
  line L6124 (77.47, 5.715) -> (76.962, 5.715)
  arc A3661 (77.216, 5.334) -> (77.216, 6.096) centre (77.216, 5.715) ccw
  arc A3662 (76.9684, 5.715) -> (77.4637, 5.715) centre (77.216, 5.715) ccw
  line L6125 (77.216, 5.969) -> (77.216, 5.461)
  arc A3663 (76.9684, 5.715) -> (77.4637, 5.715) centre (77.216, 5.715) ccw
  arc A3664 (77.216, 5.334) -> (77.216, 6.096) centre (77.216, 5.715) ccw
  arc A3665 (77.216, 6.096) -> (77.216, 5.334) centre (77.216, 5.715) ccw
  arc A3666 (85.852, 30.226) -> (85.852, 29.718) centre (85.852, 29.972) ccw
  line L6126 (92.583, 32.639) -> (94.488, 32.639)
  line L6127 (94.488, 35.179) -> (91.948, 35.179)
  line L6128 (77.47, 5.715) -> (76.962, 5.715)
  line L6129 (77.216, 5.969) -> (77.216, 5.461)
  line L6130 (92.2274, 32.9184) -> (94.2086, 32.9184)
  arc A3667 (86.36, 29.972) -> (85.344, 29.972) centre (85.852, 29.972) ccw
  arc A3668 (78.873, 22.4351) -> (78.873, 22.6129) centre (78.873, 22.524) ccw
  arc A3669 (77.273, 22.6129) -> (77.273, 22.4351) centre (77.273, 22.524) ccw
  arc A3670 (74.873, 22.4351) -> (74.873, 22.6129) centre (74.873, 22.524) ccw
  arc A3671 (78.073, 22.6129) -> (78.073, 22.4351) centre (78.073, 22.524) ccw
  arc A3672 (76.473, 22.6129) -> (76.473, 22.4351) centre (76.473, 22.524) ccw
  arc A3673 (75.673, 22.6129) -> (75.673, 22.4351) centre (75.673, 22.524) ccw
  line L6131 (92.71, 35.4076) -> (93.726, 35.4076)
  arc A3674 (74.873, 22.4351) -> (74.873, 22.6129) centre (74.873, 22.524) ccw
  arc A3675 (77.273, 22.6129) -> (77.273, 22.4351) centre (77.273, 22.524) ccw
  arc A3676 (79.673, 22.4351) -> (79.673, 22.6129) centre (79.673, 22.524) ccw
  arc A3677 (75.673, 22.6129) -> (75.673, 22.4351) centre (75.673, 22.524) ccw
  arc A3678 (75.673, 22.6129) -> (75.673, 22.4351) centre (75.673, 22.524) ccw
  arc A3679 (75.673, 22.4351) -> (75.673, 22.6129) centre (75.673, 22.524) ccw
  arc A3680 (74.873, 22.6129) -> (74.873, 22.4351) centre (74.873, 22.524) ccw
  arc A3681 (78.073, 22.4351) -> (78.073, 22.6129) centre (78.073, 22.524) ccw
  arc A3682 (74.073, 22.4351) -> (74.073, 22.6129) centre (74.073, 22.524) ccw
  line L6132 (94.7166, 32.8041) -> (94.7166, 35.0139)
  arc A3683 (80.473, 22.4351) -> (80.473, 22.6129) centre (80.473, 22.524) ccw
  arc A3684 (78.073, 22.4351) -> (78.073, 22.6129) centre (78.073, 22.524) ccw
  line L6133 (92.71, 35.4076) -> (93.726, 35.4076)
  arc A3685 (77.273, 22.4351) -> (77.273, 22.6129) centre (77.273, 22.524) ccw
  arc A3686 (80.473, 22.6129) -> (80.473, 22.4351) centre (80.473, 22.524) ccw
  arc A3687 (74.073, 22.6129) -> (74.073, 22.4351) centre (74.073, 22.524) ccw
  arc A3688 (74.873, 22.6129) -> (74.873, 22.4351) centre (74.873, 22.524) ccw
  arc A3689 (74.073, 22.6129) -> (74.073, 22.4351) centre (74.073, 22.524) ccw
  arc A3690 (78.073, 22.6129) -> (78.073, 22.4351) centre (78.073, 22.524) ccw
  arc A3691 (73.273, 22.4351) -> (73.273, 22.6129) centre (73.273, 22.524) ccw
  arc A3692 (80.473, 23.4129) -> (80.473, 23.2351) centre (80.473, 23.324) ccw
  arc A3693 (79.673, 22.4351) -> (79.673, 22.6129) centre (79.673, 22.524) ccw
  arc A3694 (77.273, 22.4351) -> (77.273, 22.6129) centre (77.273, 22.524) ccw
  arc A3695 (77.273, 22.6129) -> (77.273, 22.4351) centre (77.273, 22.524) ccw
  arc A3696 (78.073, 22.6129) -> (78.073, 22.4351) centre (78.073, 22.524) ccw
  arc A3697 (76.473, 22.4351) -> (76.473, 22.6129) centre (76.473, 22.524) ccw
  arc A3698 (74.073, 22.4351) -> (74.073, 22.6129) centre (74.073, 22.524) ccw
  line L6134 (81.473, 32.324) -> (81.473, 21.524)
  arc A3699 (78.073, 22.4351) -> (78.073, 22.6129) centre (78.073, 22.524) ccw
  arc A3700 (73.273, 22.6129) -> (73.273, 22.4351) centre (73.273, 22.524) ccw
  arc A3701 (74.873, 22.4351) -> (74.873, 22.6129) centre (74.873, 22.524) ccw
  arc A3702 (77.273, 22.4351) -> (77.273, 22.6129) centre (77.273, 22.524) ccw
  arc A3703 (79.673, 22.6129) -> (79.673, 22.4351) centre (79.673, 22.524) ccw
  line L6135 (92.71, 32.4104) -> (93.726, 32.4104)
  arc A3704 (80.473, 22.6129) -> (80.473, 22.4351) centre (80.473, 22.524) ccw
  arc A3705 (78.873, 22.4351) -> (78.873, 22.6129) centre (78.873, 22.524) ccw
  arc A3706 (79.673, 22.6129) -> (79.673, 22.4351) centre (79.673, 22.524) ccw
  arc A3707 (76.473, 22.6129) -> (76.473, 22.4351) centre (76.473, 22.524) ccw
  arc A3708 (76.473, 22.6129) -> (76.473, 22.4351) centre (76.473, 22.524) ccw
  line L6136 (70.673, 32.324) -> (81.473, 32.324)
  arc A3709 (75.673, 22.4351) -> (75.673, 22.6129) centre (75.673, 22.524) ccw
  arc A3710 (82.3939, 21.984) -> (81.9321, 21.984) centre (82.163, 21.984) ccw
  arc A3711 (74.073, 22.6129) -> (74.073, 22.4351) centre (74.073, 22.524) ccw
  line L6137 (81.473, 21.524) -> (70.673, 21.524)
  arc A3712 (81.9321, 21.984) -> (82.3939, 21.984) centre (82.163, 21.984) ccw
  arc A3713 (79.673, 22.4351) -> (79.673, 22.6129) centre (79.673, 22.524) ccw
  arc A3714 (78.873, 22.6129) -> (78.873, 22.4351) centre (78.873, 22.524) ccw
  line L6138 (91.7194, 32.8041) -> (91.7194, 35.0139)
  line L6139 (94.7166, 32.8041) -> (94.7166, 35.0139)
  arc A3715 (75.673, 22.4351) -> (75.673, 22.6129) centre (75.673, 22.524) ccw
  arc A3716 (74.073, 22.4351) -> (74.073, 22.6129) centre (74.073, 22.524) ccw
  arc A3717 (76.473, 22.4351) -> (76.473, 22.6129) centre (76.473, 22.524) ccw
  line L6140 (92.71, 32.4104) -> (93.726, 32.4104)
  arc A3718 (78.873, 22.6129) -> (78.873, 22.4351) centre (78.873, 22.524) ccw
  arc A3719 (80.473, 22.4351) -> (80.473, 22.6129) centre (80.473, 22.524) ccw
  arc A3720 (74.873, 22.6129) -> (74.873, 22.4351) centre (74.873, 22.524) ccw
  arc A3721 (76.473, 22.4351) -> (76.473, 22.6129) centre (76.473, 22.524) ccw
  arc A3722 (73.273, 22.6129) -> (73.273, 22.4351) centre (73.273, 22.524) ccw
  arc A3723 (78.873, 23.2351) -> (78.873, 23.4129) centre (78.873, 23.324) ccw
  arc A3724 (73.273, 23.2351) -> (73.273, 23.4129) centre (73.273, 23.324) ccw
  arc A3725 (72.473, 22.4351) -> (72.473, 22.6129) centre (72.473, 22.524) ccw
  arc A3726 (75.673, 23.4129) -> (75.673, 23.2351) centre (75.673, 23.324) ccw
  arc A3727 (79.673, 23.4129) -> (79.673, 23.2351) centre (79.673, 23.324) ccw
  arc A3728 (78.073, 23.2351) -> (78.073, 23.4129) centre (78.073, 23.324) ccw
  arc A3729 (77.273, 23.4129) -> (77.273, 23.2351) centre (77.273, 23.324) ccw
  arc A3730 (77.273, 23.2351) -> (77.273, 23.4129) centre (77.273, 23.324) ccw
  arc A3731 (71.673, 22.6129) -> (71.673, 22.4351) centre (71.673, 22.524) ccw
  arc A3732 (80.473, 23.4129) -> (80.473, 23.2351) centre (80.473, 23.324) ccw
  arc A3733 (75.673, 23.2351) -> (75.673, 23.4129) centre (75.673, 23.324) ccw
  arc A3734 (74.873, 23.4129) -> (74.873, 23.2351) centre (74.873, 23.324) ccw
  arc A3735 (74.873, 23.2351) -> (74.873, 23.4129) centre (74.873, 23.324) ccw
  arc A3736 (74.073, 23.4129) -> (74.073, 23.2351) centre (74.073, 23.324) ccw
  arc A3737 (74.873, 23.2351) -> (74.873, 23.4129) centre (74.873, 23.324) ccw
  arc A3738 (71.673, 22.4351) -> (71.673, 22.6129) centre (71.673, 22.524) ccw